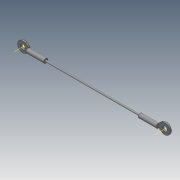
# Autodesk Inventor part: Standard
Saved by Autodesk Inventor 2020.4 (Build 244396000, 396)
## iProperties
RuleStatus: InUse
AfterDocSave0: file://Part Number Cleaner
Created: 2022-09-12
Material: Generic
Catalog Web Link: https://www.janelia.org/
Vendor: HHMI: JRC - jET
Document SubType Name: Modeling
Designer: arnoldj
Density: 1 g/cm^3
Appearance: Default
DESIGN DEPARTMENT: HHMI: JRC - jET
ALTERED ITEM PART NUMBER: N/A
ALTERED ITEM VENDOR: N/A
ALTERED ITEM DESCRIPTION: N/A
Title: Standard
Author: arnoldj
Revision Number: 0
Autodesk Inventor part; units mm, degrees
ref_plane "XZ Plane" through (0, 0, 0) normal (0, 1, 0) x (-1, 0, 0)
sketch "Sketch1" plane through (0, 0, 0) normal (0, 0, 1) x (1, 0, 0)
  line L0 (0, 7.8788) -> (0, -7.8788) projected
  line L1 (-8.0232, 0) -> (8.7455, 0) projected
  circle A0 centre (0, 0) radius 2.5797
  circle A1 centre (0, 0) radius 5.6277
  line L2 (3.1119, 4.689) -> (6.35, 2.54)
  line L3 (6.35, 2.54) -> (6.35, -2.54)
  line L4 (6.35, -2.54) -> (3.1119, -4.689)
  dimension "d0" = 5.1594
  dimension "d1" = 3.048
  dimension "d8" = 6.35
  dimension "d9" = 5.08
  constraints: 6 end point, 2 centre point, 2 coincident, 2 point on circle, 2 tangent, 1 equal length, 1 vertical
  measures "d0" diameter of A0
  measures "d1" radial gap between concentric circles of A1 A0
  measures "d8" distance between parallel lines of L3 L0
  measures "d9" distance of L2.end L3.end
extrude "Extrusion1" add sketch "Sketch1" along normal blind 1.5875 contours A1 L1 A0 L0 | L0 A0 L1 A1 | L2 L3 L1 A1 | L1 A0 L0 A1 | L1 A1 L0 A0 | L1 L3 L4 A1
sketch "Sketch2" plane through (0, 0, 0) normal (1, 0, 0) x (0, 1, 0)
  point P0 (0, 0)
ref_plane "Work Plane1" through (25.4, 0, 0) normal (1, 0, 0) x (0, 1, 0)
sketch "Sketch3" plane through (25.4, 0, 0) normal (1, 0, 0) x (0, 1, 0)
  circle A0 centre (0, 2.3495) radius 2.3495
  circle A1 centre (0, 2.3495) radius 0.762
  line L0 (5.6277, 1.5875) -> (-5.6277, 1.5875) projected
  point P0 (0, 0)
  dimension "d5" = 1.524
  constraints: 1 centre point, 1 coincident, 1 tangent, 1 vertical alignment, 2 other
  measures "d5" diameter of A1
extrude "Extrusion2" add sketch "Sketch3" against normal blind 19.05 contours A1 | A0 L0 | L0 A0
fillet "Fillet1" radius 2.54 2 edges at (6.35, 2.54, 0.7937) (6.35, -2.54, 0.7937)
sketch "Sketch4" plane through (25.4, 0, 0) normal (1, 0, 0) x (0, 1, 0)
  circle A0 centre (0, 2.3495) radius 2.3495 projected
  circle A1 centre (0, 2.3495) radius 0.889
  point P0 (0, 0)
  dimension "d11" = 1.778
  constraints: 1 centre point, 1 coincident, 1 vertical alignment
  measures "d11" diameter of A1
ref_plane "Work Plane2" through (76.2, 0, 0) normal (1, 0, 0) x (0, 1, 0)
extrude "Extrusion3" add sketch "Sketch4" along normal up to surface (50.8 mm away) contours A1
mirror "Mirror1" about plane through (76.2, 0, 0) normal (1, 0, 0) of "Extrusion3", "Extrusion2", "Fillet1", "Extrusion1"
body "Solid1"
